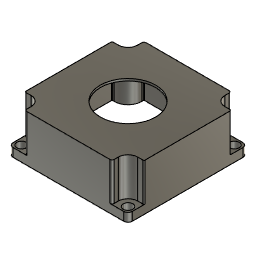
Cache_camera_ameliore v5 (Autodesk Fusion 360 design; units mm, degrees)
Autodesk Fusion 360 part; units mm, degrees
sketch "Esquisse1" plane through (0, 0, 0) normal (0, 0, 1) x (1, 0, 0)
  circle A0 centre (0, 0) radius 2.25
  line L0 (5.5, -3) -> (25, -3)
  line L1 (25, -3) -> (25, 25) construction
  line L2 (25, 25) -> (-3, 25) construction
  line L3 (-3, 25) -> (-3, 5)
  arc A1 (-3, -1) -> (-1, -3) centre (-1, -1) ccw
  line L4 (-1, 4.5) -> (0, 4.5)
  line L5 (4.5, 0) -> (4.5, -1)
  line L6 (-1, 25) -> (-1, 6.75)
  line L7 (6.76, -1) -> (25, -1)
  arc A2 (4.5, 0) -> (0, 4.5) centre (0, 0) ccw
  line L8 (-0.75, 6.5) -> (0, 6.5)
  line L9 (6.5, 0) -> (6.5, -0.74)
  arc A3 (6.5, 0) -> (0, 6.5) centre (0, 0) ccw
  line L10 (-2.5, 4.5) -> (-1, 4.5)
  line L11 (4.5, -1) -> (4.5, -2)
  arc A4 (6.5, -0.74) -> (6.76, -1) centre (6.76, -0.74) ccw
  arc A5 (-1, 6.75) -> (-0.75, 6.5) centre (-0.75, 6.75) ccw
  arc A6 (4.5, -2) -> (5.5, -3) centre (5.5, -2) ccw
  line L12 (-1, -3) -> (5.5, -3)
  arc A7 (-3, 5) -> (-2.5, 4.5) centre (-2.5, 5) ccw
  line L13 (-3, -1) -> (-3, 5)
  line L14 (45.5, -1) -> (45.5, -2)
  line L15 (53, -1) -> (53, 5)
  line L16 (51, 4.5) -> (50, 4.5)
  line L17 (52.5, 4.5) -> (51, 4.5)
  line L18 (50.75, 6.5) -> (50, 6.5)
  arc A8 (44.5, -3) -> (45.5, -2) centre (44.5, -2) ccw
  arc A9 (50, 4.5) -> (45.5, 0) centre (50, 0) ccw
  line L19 (43.24, -1) -> (25, -1)
  circle A10 centre (50, 0) radius 2.25
  line L20 (51, -3) -> (44.5, -3)
  line L21 (45.5, 0) -> (45.5, -1)
  line L22 (44.5, -3) -> (25, -3)
  arc A11 (52.5, 4.5) -> (53, 5) centre (52.5, 5) ccw
  line L23 (53, 25) -> (53, 5)
  line L24 (51, 25) -> (51, 6.75)
  arc A12 (43.24, -1) -> (43.5, -0.74) centre (43.24, -0.74) ccw
  arc A13 (50.75, 6.5) -> (51, 6.75) centre (50.75, 6.75) ccw
  line L25 (43.5, 0) -> (43.5, -0.74)
  arc A14 (51, -3) -> (53, -1) centre (51, -1) ccw
  arc A15 (50, 6.5) -> (43.5, 0) centre (50, 0) ccw
  line L26 (6.76, 51) -> (25, 51)
  arc A16 (-1, 53) -> (-3, 51) centre (-1, 51) ccw
  line L27 (53, 25) -> (53, 45)
  arc A17 (51, 43.25) -> (50.75, 43.5) centre (50.75, 43.25) ccw
  line L28 (52.5, 45.5) -> (51, 45.5)
  line L29 (45.5, 50) -> (45.5, 51)
  arc A18 (5.5, 53) -> (4.5, 52) centre (5.5, 52) ccw
  line L30 (-1, 53) -> (5.5, 53)
  line L31 (43.24, 51) -> (25, 51)
  arc A19 (53, 51) -> (51, 53) centre (51, 51) ccw
  line L32 (50.75, 43.5) -> (50, 43.5)
  line L33 (5.5, 53) -> (25, 53)
  line L34 (44.5, 53) -> (25, 53)
  line L35 (51, 45.5) -> (50, 45.5)
  arc A20 (-0.75, 43.5) -> (-1, 43.25) centre (-0.75, 43.25) ccw
  arc A21 (0, 45.5) -> (4.5, 50) centre (0, 50) ccw
  line L36 (4.5, 50) -> (4.5, 51)
  line L37 (-1, 25) -> (-1, 43.25)
  line L38 (4.5, 51) -> (4.5, 52)
  line L39 (6.5, 50) -> (6.5, 50.74)
  line L40 (51, 25) -> (51, 43.25)
  line L41 (-1, 45.5) -> (0, 45.5)
  line L42 (51, 53) -> (44.5, 53)
  line L43 (45.5, 51) -> (45.5, 52)
  arc A22 (43.5, 50.74) -> (43.24, 51) centre (43.24, 50.74) ccw
  arc A23 (53, 45) -> (52.5, 45.5) centre (52.5, 45) ccw
  arc A24 (0, 43.5) -> (6.5, 50) centre (0, 50) ccw
  line L44 (53, 51) -> (53, 45)
  arc A25 (6.76, 51) -> (6.5, 50.74) centre (6.76, 50.74) ccw
  line L45 (-3, 25) -> (-3, 45)
  arc A26 (45.5, 52) -> (44.5, 53) centre (44.5, 52) ccw
  arc A27 (43.5, 50) -> (50, 43.5) centre (50, 50) ccw
  circle A28 centre (0, 50) radius 2.25
  line L46 (43.5, 50) -> (43.5, 50.74)
  circle A29 centre (50, 50) radius 2.25
  line L47 (-0.75, 43.5) -> (0, 43.5)
  line L48 (-3, 51) -> (-3, 45)
  arc A30 (45.5, 50) -> (50, 45.5) centre (50, 50) ccw
  arc A31 (-2.5, 45.5) -> (-3, 45) centre (-2.5, 45) ccw
  line L49 (-2.5, 45.5) -> (-1, 45.5)
  circle A32 centre (25, 25) radius 13
  point P0 (50, 0)
  point P1 (25, 25)
  point P2 (25, 25)
  point P3 (25, 25)
  point P4 (0, 50)
  point P5 (50, 50)
  dimension "d22" = 4.5
  dimension "d23" = 3
  dimension "d24" = 3
  dimension "d25" = 2
  dimension "d30" = 25
  dimension "d31" = 25
  dimension "d32" = 2
  dimension "d33" = 2
  dimension "d34" = 4.5
  dimension "d35" = 4.5
  dimension "d36" = 4.5
  dimension "d37" = 2
  dimension "d38" = 2
  dimension "d39" = 6.5
  dimension "d40" = 0.26
  dimension "d41" = 0.25
  dimension "d42" = 1
  dimension "d43" = 0.5
  dimension "d44" = 26
  constraint coincident A0.centre A2.centre
  constraint horizontal L0
  constraint vertical L1
  constraint horizontal L2
  constraint vertical L3
  constraint tangent L0 A1
  constraint tangent L3 A1
  constraint perpendicular L3 L4
  constraint perpendicular L4 L5
  constraint coincident L2 L6.start
  constraint perpendicular L4 L6
  constraint perpendicular L5 L7
  constraint tangent L4 A2
  constraint tangent L5 A2
  constraint perpendicular L6 L8
  constraint perpendicular L8 L9
  constraint tangent L8 A3
  constraint tangent L9 A3
  constraint perpendicular L6 L10
  constraint perpendicular L0 L11
  constraint tangent L9 A4
  constraint tangent L7 A4
  constraint tangent L8 A5
  constraint tangent L6 A5
  constraint coincident L0 A1.end
  constraint tangent L0 A6
  constraint tangent L11 A6
  constraint coincident L3 A1.start
  constraint tangent L10 A7
  constraint tangent L3 A7
  constraint symmetric A0.centre L1 A9.centre
  constraint symmetric A0 L1 A10
  constraint symmetric L0.end L1 L22.end
  constraint symmetric P2 L1 P1
  constraint symmetric L2.end L1 L23.start
  constraint symmetric L1 A1.end L20.start
  constraint symmetric L1 A1.start L15.start
  constraint symmetric L1 A1 A14
  constraint symmetric L1 L4.start L16.start
  constraint symmetric L1 L5.end L14.start
  constraint symmetric L1 L6.start L24.start
  constraint symmetric L1 L7.end L19.end
  constraint symmetric L1 L4.end L16.end
  constraint symmetric L1 L5.start A9.end
  constraint symmetric L1 A2 A9
  constraint symmetric L1 L8.end L18.end
  constraint symmetric L1 L9.start L25.start
  constraint symmetric L1 A3 A15
  constraint symmetric L1 L9.end A12.end
  constraint symmetric L1 L7.start L19.start
  constraint symmetric L1 A4 A12
  constraint symmetric L1 L8.start L18.start
  constraint symmetric L1 L6.end L24.end
  constraint symmetric L1 A5 A13
  constraint symmetric L1 L0.start A8.start
  constraint symmetric L1 L11.end L14.end
  constraint symmetric L1 A6 A8
  constraint symmetric L1 L10.start L17.start
  constraint symmetric L1 L3.end L15.end
  constraint symmetric L1 A7 A11
  constraint symmetric A0.centre L2 P4
  constraint symmetric A0 L2 A28
  constraint symmetric L0.end L2 L33.end
  constraint symmetric P2 L2 P1
  constraint symmetric L3.start L2 L45.start
  constraint symmetric L2 A1.end A16.start
  constraint symmetric L2 A1.start A16.end
  constraint symmetric L2 A1 A16
  constraint symmetric L2 L4.start L41.start
  constraint symmetric L2 L5.end L36.end
  constraint symmetric L2 L6.start L37.start
  constraint symmetric L2 L7.end L26.end
  constraint symmetric L2 L4.end A21.start
  constraint symmetric L2 L5.start A21.end
  constraint symmetric L2 A2 A21
  constraint symmetric L2 L8.end A24.start
  constraint symmetric L2 L9.start L39.start
  constraint symmetric L2 A3 A24
  constraint symmetric L2 L9.end L39.end
  constraint symmetric L2 L7.start L26.start
  constraint symmetric L2 A4 A25
  constraint symmetric L2 L8.start A20.start
  constraint symmetric L2 L6.end A20.end
  constraint symmetric L2 A5 A20
  constraint symmetric L2 L0.start A18.start
  constraint symmetric L2 L11.end A18.end
  constraint symmetric L2 A6 A18
  constraint symmetric L2 L10.start A31.start
  constraint symmetric L2 L3.end L45.end
  constraint symmetric L2 A7 A31
  constraint symmetric L2 L20.start A19.end
  constraint symmetric L2 L0.end L33.end
  constraint symmetric L2 L15.start A19.start
  constraint symmetric L2 P0 P5
  constraint symmetric L2 P3 P2
  constraint symmetric L2 L23.start L27.start
  constraint symmetric L2 L24.start L40.start
  constraint symmetric L2 L16.end L35.end
  constraint symmetric L2 L17.start L28.start
  constraint symmetric L2 L14.end L43.end
  constraint symmetric L2 L18.start A17.end
  constraint symmetric L2 L18.end L32.end
  constraint symmetric L2 A8.start L34.start
  constraint symmetric L2 L25.start A27.start
  constraint symmetric L2 A9.end L29.start
  constraint symmetric L2 L24.end A17.start
  constraint symmetric L2 L14.start L29.end
  constraint symmetric L2 L15.end L27.end
  constraint symmetric L2 L19.start L31.start
  constraint symmetric L2 A12.end A22.start
  constraint symmetric L2 L16.start L28.end
  constraint symmetric L2 A8 A26
  constraint symmetric L2 A9 A30
  constraint symmetric L2 A10 A29
  constraint symmetric L2 A11 A23
  constraint symmetric L2 A12 A22
  constraint symmetric L2 A13 A17
  constraint symmetric L2 A14 A19
  constraint symmetric L2 A15 A27
  constraint coincident P3 P2
  measures "d22" diameter of A0
  measures "d23" distance of A0.centre L3
  measures "d24" distance of A0.centre L0
  measures "d25" radius of A1
  measures "d30" distance of A0.centre L1
  measures "d31" distance of A0.centre L2
  measures "d32" distance of L3 L6
  measures "d33" distance of L0 L7
  measures "d34" distance of A0.centre L4
  measures "d35" distance of A0.centre L5
  measures "d36" radius of A2
  measures "d37" distance of L4 L8
  measures "d38" distance of L5 L9
  measures "d39" radius of A3
  measures "d40" radius of A4
  measures "d41" radius of A5
  measures "d42" radius of A6
  measures "d43" radius of A7
  measures "d44" diameter of A32
extrude "Extrusion1" add sketch "Esquisse1" along normal blind 4 contours L0 L3 L4 L5 A2 L10 L11 A6 A7 L14 L16 L17 A8 A9 L21 L22 A11 L23 L27 L28 L29 A18 L33 L34 L35 A21 L36 L38 L41 L43 A23 L45 A26 A30 A31 L49 | A1 L4 L5 A2 L10 L11 A6 L12 A7 L13 | L14 L15 L16 L17 A8 A9 L20 L21 A11 A14 | A16 A18 L30 A21 L36 L38 L41 L48 A31 L49 | L28 L29 A19 L35 L42 L43 A23 L44 A26 A30
extrude "Extrusion2" add sketch "Esquisse1" along normal blind 16.9 from surface at 4 contours L0 L3 L4 L5 A2 L10 L11 A6 A7 L14 L16 L17 A8 A9 L21 L22 A11 L23 L27 L28 L29 A18 L33 L34 L35 A21 L36 L38 L41 L43 A23 L45 A26 A30 A31 L49
extrude "Extrusion3" add sketch "Esquisse1" along normal blind 1 from surface at 20.9 contours L0 L3 L4 L5 A2 L10 L11 A6 A7 L14 L16 L17 A8 A9 L21 L22 A11 L23 L27 L28 L29 A18 L33 L34 L35 A21 L36 L38 L41 L43 A23 L45 A26 A30 A31 L49 | L6 L7 L8 L9 A3 A4 A5 L18 L19 L24 A12 A13 L25 A15 L26 A17 L31 L32 A20 L37 L39 L40 A22 A24 A25 A27 L46 L47
equation "d48 = 8.9 mm + 8 mm"
equation "d50 = 12.9 mm + 8 mm"
